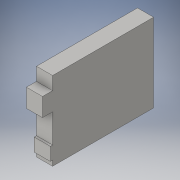
# Autodesk Inventor part: msheehan_uno_board
Saved by Autodesk Inventor 2016 (Build 200138000, 138)
## iProperties
Created: 2017-09-12
Part Number: msheehan_uno_board
Material: Generic
Document SubType Name: Modeling
Designer: Student
Density: 1 g/cm^3
Appearance: Default
Author: Student
Autodesk Inventor part; units mm, degrees
ref_plane "YZ Plane" through (0, 0, 0) normal (1, 0, 0) x (0, 1, 0)
ref_plane "XZ Plane" through (0, 0, 0) normal (0, 1, 0) x (-1, 0, 0)
ref_plane "XY Plane" through (0, 0, 0) normal (0, 0, 1) x (1, 0, 0)
sketch "Sketch1" plane through (0, 0, 0) normal (1, 0, 0) x (0, 1, 0)
  line L0 (53.34, 0) -> (53.34, -68.58)
  line L1 (53.34, -68.58) -> (0, -68.58)
  line L2 (0, -68.58) -> (0, 0)
  line L3 (53.34, 0) -> (44.45, 0)
  line L4 (44.45, 0) -> (44.45, 6.858)
  line L5 (44.45, 6.858) -> (32.004, 6.858)
  line L6 (32.004, 6.858) -> (32.004, 0)
  line L7 (44.45, 0) -> (53.34, 0)
  line L8 (0, 0) -> (3.6068, 0)
  line L9 (3.6068, 0) -> (3.6068, 1.524)
  line L10 (3.6068, 1.524) -> (12.4968, 1.524)
  line L11 (12.4968, 1.524) -> (12.4968, 0)
  line L12 (0, 0) -> (3.6068, 0)
  line L13 (12.4968, 0) -> (32.004, 0)
  dimension "d0" = 53.34
  dimension "d1" = 68.58
  dimension "d2" = 8.89
  dimension "d3" = 6.858
  dimension "d4" = 12.446
  dimension "d5" = 3.6068
  dimension "d6" = 1.524
  dimension "d7" = 8.89
  constraints: 28 end point, 11 perpendicular, 4 parallel, 3 horizontal, 1 vertical
  measures "d0" distance of L0.end L1.end
  measures "d1" distance of L0.start L0.end
  measures "d2" distance of L0.start L3.end
  measures "d3" distance of L3.end L4.end
  measures "d4" distance of L4.end L5.end
  measures "d5" distance of L2.end L8.end
  measures "d6" distance of L8.end L9.end
  measures "d7" distance of L9.end L10.end
extrude "Extrusion1" add sketch "Sketch1" along normal blind 10.922
body "Solid1"
